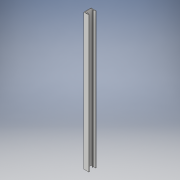
# Autodesk Inventor part: mainbar
Saved by Autodesk Inventor 2019.3 (Build 233278000, 278)
## iProperties
Created: 2019-04-14
Part Number: mainbar
Material: Generic
Document SubType Name: Modeling
Designer: peter
Density: 1 g/cm^3
Appearance: Default
Author: peter
Autodesk Inventor part; units mm, degrees
ref_plane "YZ Plane" through (0, 0, 0) normal (1, 0, 0) x (0, 1, 0)
ref_plane "XZ Plane" through (0, 0, 0) normal (0, 1, 0) x (-1, 0, 0)
ref_plane "XY Plane" through (0, 0, 0) normal (0, 0, 1) x (1, 0, 0)
sketch "Sketch1" plane through (0, 0, 0) normal (0, 1, 0) x (-1, 0, 0)
  line L0 (0, 0) -> (10.5, 0)
  line L1 (10.5, 0) -> (10.5, -15)
  line L2 (10.5, -15) -> (0, -15)
  line L3 (0, -15) -> (0, -14)
  line L4 (9.5, -14) -> (9.5, -1)
  line L5 (0, -1) -> (0, 0)
  line L6 (9.5, -1) -> (5.5, -1)
  line L7 (5.5, -1) -> (5.5, -3)
  line L8 (5.5, -3) -> (4.5, -3)
  line L9 (4.5, -3) -> (4.5, -1)
  line L10 (5.5, -14) -> (5.5, -12)
  line L11 (5.5, -12) -> (4.5, -12)
  line L12 (4.5, -12) -> (4.5, -14)
  line L13 (9.5, -1) -> (5.5, -1)
  line L14 (4.5, -1) -> (0, -1)
  line L15 (0, -14) -> (4.5, -14)
  line L16 (5.5, -14) -> (9.5, -14)
  dimension "d0" = 10.5
  dimension "d1" = 15
  dimension "d2" = 1
  dimension "d3" = 9.5
  dimension "d4" = 13
  dimension "d5" = 4
  dimension "d6" = 2
  dimension "d7" = 1
  dimension "d8" = 2
  dimension "d9" = 1
  dimension "d10" = 2
  constraints: 34 end point, 14 perpendicular, 3 point on line, 1 horizontal, 1 vertical
  measures "d0" distance of L0.start L0.end
  measures "d1" distance of L0.end L1.end
  measures "d2" distance of L2.end L3.end
  measures "d3" distance of L3.end L4.start
  measures "d4" distance of L4.start L4.end
  measures "d5" distance of L4.end L6.end
  measures "d6" distance of L6.end L7.end
  measures "d7" distance of L7.end L8.end
  measures "d8" distance of L10.start L10.end
  measures "d9" distance of L10.end L11.end
  measures "d10" distance of L11.end L12.end
extrude "Extrusion1" add sketch "Sketch1" along normal blind 275
body "Solid1"
